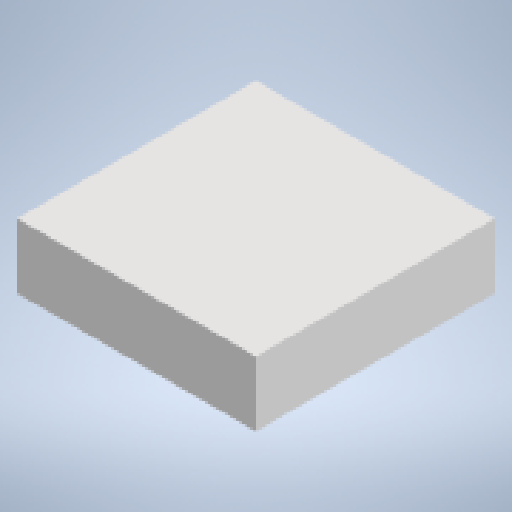
# Autodesk Inventor part: STOCK_ALUMINIO
Saved by Autodesk Inventor 2023.2 (Build 272271030, 271C)
## iProperties
Created: 2023-08-30
Part Number: STOCK_ALUMINIO
Material: Generic
Document SubType Name: Modeling
Designer: Cris Pat
Density: 1 g/cm^3
Appearance: Default
Author: Cris Pat
Autodesk Inventor part; units mm, degrees
ref_plane "YZ Plane" through (0, 0, 0) normal (1, 0, 0) x (0, 1, 0)
ref_plane "XZ Plane" through (0, 0, 0) normal (0, 1, 0) x (-1, 0, 0)
ref_plane "XY Plane" through (0, 0, 0) normal (0, 0, 1) x (1, 0, 0)
sketch "Sketch1" plane through (0, 0, 0) normal (0, 0, 1) x (1, 0, 0)
  line L0 (3, 73.2) -> (3, 3) projected
  line L1 (73.2, 73.2) -> (3, 73.2) projected
  line L2 (73.2, 3) -> (73.2, 73.2) projected
  line L3 (3, 3) -> (73.2, 3) projected
  point P0 (0, 0)
ref_plane "Work Plane1" through (-3.81, -3.81, -19.05) normal (0, 0, 1) x (1, 0, 0)
extrude "Extrusion1" add sketch "Sketch1" against normal up to surface (19.05 mm away)
body "Solid1"
